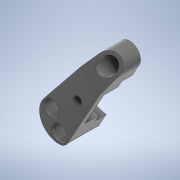
# Autodesk Inventor part: PartD_3D
Saved by Autodesk Inventor 2022 (Build 260153000, 153)
## iProperties
Created: 2021-02-22
Part Number: PartD_3D
Material: Generic
Document SubType Name: Modeling
Designer: Acer
Density: 1 g/cm^3
Appearance: Default
Author: Acer
Autodesk Inventor part; units mm, degrees
ref_plane "YZ Plane" through (0, 0, 0) normal (1, 0, 0) x (0, 1, 0)
ref_plane "XZ Plane" through (0, 0, 0) normal (0, 1, 0) x (-1, 0, 0)
ref_plane "XY Plane" through (0, 0, 0) normal (0, 0, 1) x (1, 0, 0)
sketch "Sketch1" plane through (0, 0, 0) normal (0, 0, 1) x (1, 0, 0)
  line L0 (0, 0) -> (18, 0)
  line L1 (18, 0) -> (18, 24)
  line L2 (18, 24) -> (0, 24)
  line L3 (0, 24) -> (0, 0)
  circle A0 centre (15, 21) radius 1.05
  circle A1 centre (5, 2.5) radius 1.05
  circle A2 centre (3, 7) radius 1.05
  line L4 (0, 10) -> (11.3137, 10) construction
  line L5 (6, 0) -> (28.3492, 0) construction
  line L6 (6, 0) -> (42, 0) construction
  circle A3 centre (9.749, 12) radius 1
  circle A4 centre (15, 21) radius 2.75
  circle A5 centre (5, 5) radius 5
  line L7 (1.1063, 8.1367) -> (12.8585, 22.7252)
  circle A6 centre (5, 2.5) radius 2.5
  line L8 (7.185, 1.2851) -> (17.4035, 19.6637)
  point P0 (8, 24)
  point P1 (18, 31.1769)
  point P2 (9.5257, 2.8745)
  point P3 (17.4892, 19.831)
  point P4 (5, 0)
  dimension "d0" = 18
  dimension "d1" = 24
  dimension "d2" = 2.1
  dimension "d3" = 3
  dimension "d4" = 3
  dimension "d5" = 2.1
  dimension "d6" = 2.1
  dimension "d7" = 2.5
  dimension "d8" = 5
  dimension "d9" = 3
  dimension "d10" = 7
  dimension "d12" = 10
  dimension "d15" = 6
  dimension "d18" = 2
  dimension "d25" = 5.5
  dimension "d26" = 10
  dimension "d30" = 12
  dimension "d31" = 8.251
  constraints: 18 end point, 6 centre point, 5 point on circle, 5 tangent, 4 horizontal, 4 point on line, 2 coincident, 2 parallel, 1 perpendicular, 5 other
  measures "d0" distance of L2.end L1.end
  measures "d1" distance of L1.end L0.end
  measures "d2" diameter of A0
  measures "d3" distance from line of L1 A0.centre
  measures "d4" distance from line of L2 A0.centre
  measures "d5" diameter of A1
  measures "d6" diameter of A2
  measures "d7" distance from line of A1.centre L0
  measures "d8" distance from line of L3 A1.centre
  measures "d9" distance from line of L3 A2.centre
  measures "d10" distance from line of L0 A2.centre
  measures "d12" distance of L0.start L4.start
  measures "d15" distance of L0.start L5.start
  measures "d18" diameter of A3
  measures "d25" diameter of A4
  measures "d26" diameter of A5
  measures "d30" distance from line of A3.centre L0
  measures "d31" distance from line of A3.centre L1
extrude "Extrusion1" add sketch "Sketch1" along normal blind 8 contours A5 L8 A6 | A6 | L7 A4 L8 A5 | A4 picked at (5.8937, 6.9979)
sketch "Sketch3" plane through (0, 0, 0) normal (0, 0, -1) x (-1, 0, 0)
  circle A0 centre (-9.749, 12) radius 1 projected
  circle A1 centre (-9.749, 12) radius 7.45
  point P0 (0, 0)
  dimension "d27" = 14.9
  constraints: 1 centre point, 1 coincident
  measures "d27" diameter of A1
extrude "Extrusion2" cut sketch "Sketch3" against normal blind 2.7
sketch "Sketch5" plane through (0, 0, 8) normal (0, 0, 1) x (1, 0, 0)
  circle A0 centre (3, 7) radius 1.05 projected
  circle A1 centre (5, 2.5) radius 1.05 projected
  circle A2 centre (15, 21) radius 1.05 projected
  circle A3 centre (3, 7) radius 2
  circle A4 centre (5, 2.5) radius 2
  circle A5 centre (15, 21) radius 2
  point P0 (0, 0)
  dimension "d32" = 4
  dimension "d33" = 4
  dimension "d34" = 4
  constraints: 3 centre point, 3 coincident
  measures "d32" diameter of A3
  measures "d33" diameter of A4
  measures "d34" diameter of A5
extrude "Extrusion3" cut sketch "Sketch5" against normal blind 4.9
sketch "Sketch6" plane through (0, 0, 2.7) normal (0, 0, -1) x (-1, 0, 0)
  circle A0 centre (-9.749, 12) radius 1 projected
  circle A1 centre (-9.749, 12) radius 1 projected
  circle A2 centre (-9.749, 12) radius 5.7
  point P0 (0, 0)
  dimension "d37" = 11.4
  constraints: 1 centre point, 1 coincident
  measures "d37" diameter of A2
extrude "Extrusion4" cut sketch "Sketch6" against normal blind 3.65
sketch "Sketch8" plane through (1.1063, 8.1367, 0) normal (-0.778745, 0.6273406, 0) x (0, 0, 1)
  line L0 (0, 21.4833) -> (8, 21.4833) projected
  line L1 (8, 18.7333) -> (8, 0) projected
  line L2 (8, 18.7333) -> (8, 21.4833) projected
  line L3 (4, 21.4833) -> (8, 15)
  line L4 (8, -1.5222) -> (8, 19.2005) projected
  point P0 (0, -7.0304)
  point P1 (8, 15)
  constraints: 2 end point, 1 midpoint, 1 point on line
extrude "Extrusion5" cut sketch "Sketch8" against normal up to surface surface through (7.185, 1.2851, 0) normal (0.8739914, -0.4859413, 0)
body "Solid1"
